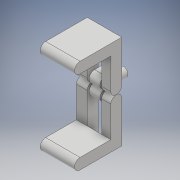
# Autodesk Inventor part: 夾爪
Saved by Autodesk Inventor 2017 (Build 210142000, 142)
## iProperties
Part Number: 夾爪
Material: 一般
Document SubType Name: Modeling
Designer: Brian
Density: 1 g/cm^3
Appearance: 預設
Author: Brian
Autodesk Inventor part; units mm, degrees
ref_plane "YZ Plane" through (0, 0, 0) normal (1, 0, 0) x (0, 1, 0)
ref_plane "XZ Plane" through (0, 0, 0) normal (0, 1, 0) x (-1, 0, 0)
sketch "草圖1" plane through (0, 0, 0) normal (0, 1, 0) x (-1, 0, 0)
  circle A0 centre (0, 0) radius 25
  dimension "d0" = 50
  constraints: 1 centre point, 1 coincident
  measures "d0" diameter of A0
extrude "擠出1" add sketch "草圖1" along normal blind 80
sketch "草圖2" plane through (0, 0, 0) normal (0, -1, 0) x (1, 0, 0)
  line L0 (30, -60) -> (-30, -60)
  line L1 (-30, -60) -> (-30, 60)
  line L2 (-30, 60) -> (30, 60)
  line L3 (30, 60) -> (30, -60)
  line L4 (30, -60) -> (-30, 60) construction
  line L5 (-30, -60) -> (30, 60) construction
  point P0 (0, 0)
  dimension "d3" = 120
  dimension "d4" = 60
  constraints: 12 end point, 2 midpoint, 2 parallel, 1 horizontal, 1 perpendicular
  measures "d3" distance of L0.end L1.end
  measures "d4" distance of L0.start L0.end
extrude "擠出2" add sketch "草圖2" along normal blind 50
sketch "草圖3" plane through (30, 0, 60) normal (1, 0, 0) x (0, 0, -1)
  line L0 (120, -50) -> (0, -50) projected
  circle A0 centre (30, -50) radius 30
  circle A1 centre (90, -50) radius 30
  point P0 (60, 0)
  dimension "d8" = 60
  dimension "d7" = 60
  constraints: 2 point on line, 1 centre point, 1 horizontal alignment, 3 other
  measures "d7" diameter of A1
extrude "擠出3" add sketch "草圖3" against normal up to surface (60 mm away)
ref_plane "工作平面1" through (40, 0, 60) normal (1, 0, 0) x (0, 0, -1)
sketch "草圖4" plane through (40, 0, 60) normal (1, 0, 0) x (0, 0, -1)
  arc A0 (0, -50) -> (60, -50) centre (30, -50) ccw projected
  line L0 (30, -50) -> (-111.4214, -191.4214)
  line L1 (-111.4214, -191.4214) -> (30, -332.8427)
  line L2 (0, 0) -> (0, -50) projected
  line L3 (51.2132, -71.2132) -> (-68.9949, -191.4214)
  line L4 (-68.9949, -191.4214) -> (51.2132, -311.6295)
  line L5 (8.7868, -28.7868) -> (-153.8478, -191.4214)
  line L6 (-153.8478, -191.4214) -> (8.7868, -354.0559)
  arc A1 (51.2132, -71.2132) -> (8.7868, -28.7868) centre (30, -50) ccw
  arc A2 (8.7868, -354.0559) -> (51.2132, -311.6295) centre (30, -332.8427) ccw
  point P0 (60, 0)
  dimension "d12" = 90
  dimension "d13" = 45
  dimension "d14" = 200
  dimension "d15" = 30
  dimension "d16" = 30
  dimension "d17" = 60
  dimension "d18" = 60
  constraints: 12 end point, 4 point on circle, 2 centre point, 2 coincident, 1 perpendicular, 2 other
  measures "d12" angle of L0 L1
  measures "d13" angle of L2 L0
  measures "d14" distance of L0.start L0.end
  measures "d15" distance between parallel lines of L0 L3
  measures "d16" distance between parallel lines of L5 L0
  measures "d17" diameter of A2
  measures "d18" diameter of A1
extrude "擠出4" add sketch "草圖4" along normal blind 50 separate body
sketch "草圖8" plane through (40, 0, 60) normal (-1, 0, 0) x (0, 0, 1)
  line L0 (-8.7868, -354.0559) -> (153.8478, -191.4214) projected
  line L1 (68.9949, -191.4214) -> (-51.2132, -311.6295) projected
  arc A0 (-51.2132, -311.6295) -> (-8.7868, -354.0559) centre (-30, -332.8427) ccw projected
  line L2 (153.8478, -191.4214) -> (-8.7868, -354.0559) projected
  line L3 (153.8478, -191.4214) -> (68.9949, -191.4214)
  point P0 (-60, 0)
  constraints: 2 end point, 1 horizontal
extrude "擠出7" add sketch "草圖8" along normal blind 80 bodies 2
sketch "草圖9" plane through (-40, 0, 60) normal (-1, 0, 0) x (0, 0, 1)
  line L0 (68.9949, -191.4214) -> (153.8478, -191.4214) projected
  line L1 (153.8478, -191.4214) -> (-8.7868, -28.7868) projected
  arc A0 (-8.7868, -28.7868) -> (-51.2132, -71.2132) centre (-30, -50) ccw projected
  line L2 (-51.2132, -71.2132) -> (68.9949, -191.4214) projected
  line L3 (-8.7868, -354.0559) -> (153.8478, -191.4214) projected
  line L4 (153.8478, -191.4214) -> (68.9949, -191.4214) projected
  line L5 (68.9949, -191.4214) -> (-51.2132, -311.6295) projected
  arc A1 (-51.2132, -311.6295) -> (-8.7868, -354.0559) centre (-30, -332.8427) ccw projected
  point P0 (-60, 0)
extrude "擠出8" add sketch "草圖9" along normal blind 60 bodies 2
move or copy body "旋轉1" bodies to move or copy 2 copy no rotation origin (0, 0, 0) rotation axis (1, 0, 0) rotation angle -45 translate (0, -35.8579, -26.5685)
mirror "鏡射1" about plane through (0, 0, 0) normal (0, 0, 1) bodies 2
